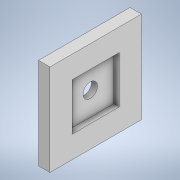
# Autodesk Inventor part: 220425 End Cap
Saved by Autodesk Inventor 2022 (Build 260153000, 153)
## iProperties
Created: 2021-11-23
Part Number: 220425 End Cap
Material: Generic
Document SubType Name: Modeling
Designer: josephinew
Density: 1 g/cm^3
Appearance: Default
Author: josephinew
Autodesk Inventor part; units mm, degrees
ref_plane "YZ Plane" through (0, 0, 0) normal (1, 0, 0) x (0, 1, 0)
ref_plane "XZ Plane" through (0, 0, 0) normal (0, 1, 0) x (-1, 0, 0)
ref_plane "XY Plane" through (0, 0, 0) normal (0, 0, 1) x (1, 0, 0)
sketch "Sketch1" plane through (0, 0, 0) normal (1, 0, 0) x (0, 1, 0)
  line L0 (0, 0) -> (50.8, 0)
  line L1 (50.8, 0) -> (50.8, -50.8)
  line L2 (50.8, -50.8) -> (0, -50.8)
  line L3 (0, -50.8) -> (0, 0)
  line L4 (50.8, 0) -> (50.8, -25.4)
  circle A0 centre (25.4, -25.4) radius 4.0132
  dimension "d0" = 50.8
  dimension "d1" = 50.8
  dimension "d5" = 8.0264
  constraints: 10 end point, 2 parallel, 1 centre point, 1 horizontal, 1 midpoint, 1 perpendicular
  measures "d0" distance of L1.end L2.end
  measures "d1" distance of L0.end L1.end
  measures "d5" diameter of A0
extrude "Extrusion1" add sketch "Sketch1" along normal blind 11.43
sketch "Sketch2" plane through (11.43, 0, 0) normal (1, 0, 0) x (0, 0, -1)
  line L0 (12.319, 38.481) -> (38.481, 38.481)
  line L1 (38.481, 38.481) -> (38.481, 12.319)
  line L2 (38.481, 12.319) -> (12.319, 12.319)
  line L3 (12.319, 12.319) -> (12.319, 38.481)
  line L4 (50.8, 50.8) -> (0, 50.8) projected
  line L5 (0, 0) -> (50.8, 0) projected
  line L6 (0, 50.8) -> (0, 0) projected
  dimension "d8" = 26.162
  dimension "d9" = 26.162
  constraints: 8 end point, 2 parallel, 1 horizontal, 1 perpendicular
  measures "d8" distance of L1.end L2.end
  measures "d9" distance of L0.end L1.end
extrude "Extrusion2" cut sketch "Sketch2" against normal blind 3.048
sketch "Sketch3" plane through (0, 0, 0) normal (-1, 0, 0) x (0, 0, 1)
  circle A0 centre (-25.4, 25.4) radius 4.0132 projected
  circle A1 centre (-25.4, 25.4) radius 8.255
  point P0 (0, 0)
  dimension "d12" = 16.51
  constraints: 1 centre point, 1 coincident
  measures "d12" diameter of A1
extrude "Extrusion3" cut sketch "Sketch3" against normal blind 1.905
sketch "Sketch4" plane through (0, 0, 0) normal (0, 0, 1) x (1, 0, 0)
  line L0 (0, 0) -> (11.43, 0) projected
  line L1 (0, 50.8) -> (11.43, 50.8) projected
  line L2 (0, 0) -> (5.08, 0)
  line L3 (5.08, 0) -> (5.08, 50.8)
  line L4 (5.08, 50.8) -> (0, 50.8)
  line L5 (0, 50.8) -> (0, 0)
  dimension "d15" = 5.08
  constraints: 8 end point, 2 parallel, 1 horizontal, 1 perpendicular, 1 point on line
  measures "d15" distance of L4.end L3.end
extrude "Extrusion4" cut sketch "Sketch4" against normal blind 50.8
body "Solid1"
